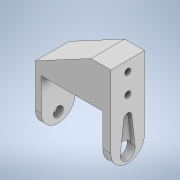
# Autodesk Inventor part: juncao6
Saved by Autodesk Inventor 2022.1 (Build 261234000, 234)
## iProperties
Created: 2021-08-04
Part Number: juncao6
Material: Generic
Document SubType Name: Modeling
Designer: nakai
Density: 1 g/cm^3
Appearance: Default
Author: nakai
Autodesk Inventor part; units mm, degrees
ref_plane "YZ Plane" through (0, 0, 0) normal (1, 0, 0) x (0, 1, 0)
ref_plane "XZ Plane" through (0, 0, 0) normal (0, 1, 0) x (-1, 0, 0)
ref_plane "XY Plane" through (0, 0, 0) normal (0, 0, 1) x (1, 0, 0)
sketch "Sketch1" plane through (0, 0, 0) normal (0, 0, 1) x (1, 0, 0)
  line L0 (0, 0) -> (3, 0)
  line L1 (3, 0) -> (3, 25)
  line L2 (3, 25) -> (0, 25)
  line L3 (0, 25) -> (0, 0)
  line L4 (34, 25) -> (38, 25)
  line L5 (38, 25) -> (38, 0)
  line L6 (38, 0) -> (34, 0)
  line L7 (34, 0) -> (34, 25)
  line L8 (0, 25) -> (38, 25)
  line L9 (38, 25) -> (38, 45)
  line L10 (38, 45) -> (0, 45)
  line L11 (0, 45) -> (0, 25)
  line L12 (0, 25) -> (0, 30)
  line L13 (0, 30) -> (28, 45)
  line L14 (28, 45) -> (38, 45)
  point P0 (34, 25)
  dimension "d0" = 3
  dimension "d1" = 25
  dimension "d2" = 4
  dimension "d3" = 25
  dimension "d4" = 31
  dimension "d5" = 38
  dimension "d6" = 20
  dimension "d7" = 5
  dimension "d10" = 10
  constraints: 30 end point, 6 parallel, 3 horizontal, 3 perpendicular, 3 point on line, 1 collinear
  measures "d0" distance of L2.end L1.end
  measures "d1" distance of L1.end L0.end
  measures "d2" distance of L5.end L6.end
  measures "d3" distance of L4.end L5.end
  measures "d4" distance between parallel lines of L7 L1
  measures "d5" distance of L10.end L9.end
  measures "d6" distance of L9.end L8.end
  measures "d7" distance of L2.end L12.end
  measures "d10" distance of L9.end L13.end
extrude "Extrusion1" add sketch "Sketch1" along normal blind 17 contours L3 L2 L1 L0 | L11 L13 L10 L9 L4 L8 L2 | L4 L5 L6 L7
sketch "Sketch2" plane through (38, 0, 0) normal (1, 0, 0) x (0, 0, -1)
  line L0 (0, 25) -> (-17, 25) projected
  line L1 (0, 0) -> (0, 45) projected
  line L2 (-17, 25) -> (0, 25)
  line L3 (0, 25) -> (0, 45)
  line L4 (0, 45) -> (-17, 45)
  line L5 (-17, 45) -> (-17, 25)
  circle A0 centre (-8.5, 30) radius 1.5
  circle A1 centre (-8.5, 40) radius 1.5
  dimension "d11" = 3
  dimension "d12" = 3
  dimension "d13" = 5
  dimension "d15" = 8.5
  dimension "d16" = 5
  dimension "d19" = 17
  dimension "d20" = 8.5
  dimension "d21" = 20
  constraints: 8 end point, 2 centre point, 2 parallel, 1 horizontal, 1 perpendicular
  measures "d11" diameter of A0
  measures "d12" diameter of A1
  measures "d13" distance from line of A0.centre L0
  measures "d15" distance from line of L5 A1.centre
  measures "d16" distance from line of L4 A1.centre
  measures "d19" distance of L0.start L0.end
  measures "d20" distance from line of L5 A0.centre
  measures "d21" distance of L4.end L0.end
extrude "Extrusion2" cut sketch "Sketch2" against normal blind 10 contours A0 | A1
sketch "Sketch3" plane through (38, 0, 0) normal (1, 0, 0) x (0, 0, -1)
  circle A0 centre (-8.5, 5) radius 3.75
  line L0 (0, 0) -> (-17, 0) projected
  line L1 (0, 0) -> (0, 45) projected
  point P0 (-8.5, 0)
  dimension "d22" = 7.5
  dimension "d23" = 5
  dimension "d24" = 8.5
  constraints: 1 centre point, 1 midpoint
  measures "d22" diameter of A0
  measures "d23" distance of point (-8.5, 0) A0.centre
  measures "d24" distance from line of L1 A0.centre
extrude "Extrusion3" cut sketch "Sketch3" against normal up to surface (4 mm away)
fillet "Fillet1" radius 8.5 4 edges at (36, 0, 17) (1.5, 0, 17) (1.5, 0, 0) (36, 0, 0)
sketch "Sketch4" plane through (0, 30, 0) normal (-1, 0, 0) x (0, 0, 1)
  circle A0 centre (8.5, -25) radius 2.5
  arc A1 (0, -21.5) -> (17, -21.5) centre (8.5, -21.5) ccw projected
  line L0 (17, 0) -> (17, -21.5) projected
  point P0 (0, -30)
  point P1 (8.5, -30)
  dimension "d28" = 5
  dimension "d29" = 5
  dimension "d30" = 8.5
  constraints: 1 centre point, 1 point on circle
  measures "d28" diameter of A0
  measures "d29" distance of A0.centre point (8.5, -30)
  measures "d30" distance from line of L0 A0.centre
extrude "Extrusion4" cut sketch "Sketch4" against normal up to surface (3 mm away)
sketch "Sketch5" plane through (38, 45, 17) normal (1, 0, 0) x (0, 0, -1)
  circle A0 centre (8.5, -40) radius 3.75 projected
  circle A1 centre (8.5, -40) radius 3.5
  circle A2 centre (8.5, -25) radius 2
  circle A3 centre (8.5, -40) radius 3.75
  line L0 (10.4863, -24.7667) -> (12.2244, -39.5625)
  line L1 (6.5137, -24.7667) -> (4.7756, -39.5625)
  point P0 (17, -45)
  dimension "d33" = 4
  dimension "d34" = 15
  dimension "d35" = 0
  constraints: 4 end point, 4 point on circle, 4 tangent, 3 centre point, 1 coincident
  measures "d33" diameter of A2
  measures "d34" distance of A3.centre A2.centre
  measures "d35" horizontal distance of A3.centre A2.centre
extrude "Extrusion5" cut sketch "Sketch5" against normal blind 2 contours A0 | A0 L1 A2 L0 | A2 | A1
body "Solid1"
